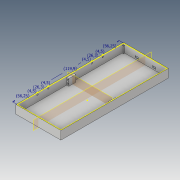
# Autodesk Inventor part: Case Board
Saved by Autodesk Inventor 2019 (Build 230136000, 136)
## iProperties
Created: 2020-09-15
Part Number: Case Board
Material: Generic
Document SubType Name: Modeling
Designer: giacomo
Density: 1 g/cm^3
Appearance: Default
Author: giacomo
Autodesk Inventor part; units mm, degrees
ref_plane "YZ Plane" through (0, 0, 0) normal (1, 0, 0) x (0, 1, 0)
ref_plane "XZ Plane" through (0, 0, 0) normal (0, 1, 0) x (-1, 0, 0)
ref_plane "XY Plane" through (0, 0, 0) normal (0, 0, 1) x (1, 0, 0)
sketch "Sketch1" plane through (0, 0, 0) normal (0, 1, 0) x (-1, 0, 0)
  line L0 (80.1493, 105.9266) -> (-24.8507, 105.9266) construction
  line L1 (-24.8507, 105.9266) -> (-24.8507, -189.0734) construction
  line L2 (-24.8507, -189.0734) -> (80.1493, -189.0734) construction
  line L3 (80.1493, -189.0734) -> (80.1493, 105.9266) construction
  line L4 (80.1493, 91.9266) -> (83.1493, 91.9266) construction
  line L5 (83.1493, 91.9266) -> (83.1493, 84.3266) construction
  line L6 (83.1493, 84.3266) -> (80.1493, 84.3266) construction
  line L7 (80.1493, 84.3266) -> (80.1493, 91.9266) construction
  point P0 (0, 0)
  dimension "d0" = 295
  dimension "d1" = 105
  dimension "d2" = 7.6
  dimension "d3" = 3
  dimension "d4" = 14
  constraints: 16 end point, 4 parallel, 2 horizontal, 2 perpendicular, 1 point on line
  measures "d0" distance of L2.end L0.start
  measures "d1" distance of L1.end L2.end
  measures "d2" distance of L4.end L5.end
  measures "d3" distance of L5.end L6.end
  measures "d4" distance between parallel lines of L0 L4
sketch "Sketch2" plane through (0, 0, 0) normal (0, 1, 0) x (-1, 0, 0)
  line L0 (80.1493, -189.0734) -> (80.1493, 105.9266) construction
  line L1 (-24.8507, -189.0734) -> (80.1493, -189.0734) construction
  line L2 (-24.8507, 105.9266) -> (-24.8507, -189.0734) construction
  line L3 (80.1493, 105.9266) -> (-24.8507, 105.9266) construction
  line L4 (90.1493, 109.9266) -> (90.1493, -193.0734)
  line L5 (-34.8507, -193.0734) -> (-34.8507, 109.9266)
  line L6 (90.1493, 109.9266) -> (-34.8507, 109.9266)
  line L7 (90.1493, -193.0734) -> (-34.8507, -193.0734)
  line L8 (91.6493, -194.5734) -> (91.6493, 111.4266)
  line L9 (91.6493, 111.4266) -> (-36.3507, 111.4266)
  line L10 (-36.3507, 111.4266) -> (-36.3507, -194.5734)
  line L11 (-36.3507, -194.5734) -> (91.6493, -194.5734)
  dimension "d71" = 10
  dimension "d72" = 4
  dimension "d73" = 10
  dimension "d74" = 4
  dimension "d75" = 1.5
  constraints: 16 end point, 2 parallel, 2 perpendicular, 3 other
  measures "d71" distance between parallel lines of L0 L4
  measures "d72" distance between parallel lines of L6 L3
  measures "d73" distance between parallel lines of L2 L5
  measures "d74" distance between parallel lines of L1 L7
  measures "d75" distance between parallel lines of L4 L8
extrude "Extrusion1" add sketch "Sketch2" against normal blind 1 contours L4 L7 L5 L6
extrude "Extrusion2" add sketch "Sketch2" along normal blind 23 and the other way blind 1
sketch "Sketch5" plane through (-91.6493, -1, 111.4266) normal (-1, 0, 0) x (0, 0, 1)
  circle A0 centre (-246, 19) radius 2.25
  circle A1 centre (-90.8, 19) radius 2.25
  circle A2 centre (-215.2, 19) radius 2.25
  circle A3 centre (-60, 19) radius 2.25
  line L0 (0, 0) -> (0, 24) projected
  line L1 (-306, 24) -> (0, 24) projected
  line L2 (-306, 24) -> (-306, 0) projected
  line L3 (0, 0) -> (-306, 0) projected
  point P0 (-111.4266, 1)
  dimension "d35" = 4.5
  dimension "d37" = 4.5
  dimension "d39" = 4.5
  dimension "d40" = 0
  dimension "d41" = 30.8
  dimension "d45" = 4.5
  dimension "d46" = 0
  dimension "d47" = 30.8
  dimension "d76" = 60
  dimension "d77" = 60
  dimension "d144" = 5
  dimension "d145" = 5
  constraints: 4 centre point
  measures "d35" diameter of A0
  measures "d37" diameter of A1
  measures "d39" diameter of A2
  measures "d40" vertical distance of A2.centre A0.centre
  measures "d41" distance of A2.centre A0.centre
  measures "d45" diameter of A3
  measures "d46" vertical distance of A3.centre A1.centre
  measures "d47" distance of A3.centre A1.centre
  measures "d76" distance from line of L2 A0.centre
  measures "d77" distance from line of L0 A3.centre
  measures "d144" distance from line of L1 A2.centre
  measures "d145" distance from line of L1 A1.centre
extrude "Extrusion4" cut sketch "Sketch5" against normal up to surface (1.5 mm away) contours A0 | A1 | A2 | A3
sketch "Sketch7" plane through (-90.1493, 0, -193.0734) normal (1, 0, 0) x (0, 0, -1)
  line L0 (-151.5, 23) -> (-151.5, 0) construction
  line L1 (-141.5, 19) -> (-141.5, 0)
  line L2 (-161.5, 19) -> (-161.5, 0)
  line L3 (-303, 23) -> (0, 23) projected
  line L4 (-303, 0) -> (0, 0) projected
  line L5 (0, 23) -> (0, 0) projected
  line L6 (-161.5, 19) -> (-141.5, 19)
  point P0 (-141.5, 23)
  point P1 (-161.5, 23)
  dimension "d106" = 10
  dimension "d107" = 10
  dimension "d148" = 151.5
  dimension "d149" = 151.5
  dimension "d193" = 19
  constraints: 8 end point, 1 perpendicular
  measures "d106" distance between parallel lines of L1 L0
  measures "d107" distance between parallel lines of L2 L0
  measures "d148" distance from line of L3.start L0
  measures "d149" distance between parallel lines of L5 L0
  measures "d193" distance between parallel lines of L4 L6
extrude "Extrusion6" add sketch "Sketch7" along normal blind 6
ref_plane "Work Plane2" through (-27.6493, 0, 109.9266) normal (1, 0, 0) x (0, 0, -1)
ref_plane "Work Plane4" through (-90.1493, 0, -41.5734) normal (0, 0, 1) x (1, 0, 0)
sketch "Sketch16" plane through (-90.1493, 0, -31.5734) normal (0, 0, 1) x (1, 0, 0)
  line L0 (0, 0) -> (0, 19) projected
  line L1 (0, 19) -> (6, 19) projected
  point P0 (90.1493, 0)
  point P1 (3.5, 14)
  dimension "d108" = 3.5
  dimension "d194" = 5
  measures "d108" distance from line of L0 point (3.5, 14)
  measures "d194" distance from line of L1 point (3.5, 14)
hole "Hole3" at (-86.6493, 14, -31.5734) direction (0, 0, -1) diameter 2.6 depth 5 countersink diameter 5 countersink angle 82
sketch "Sketch17" plane through (-86.6493, 14, -36.5734) normal (0, 0, 1) x (1, 0, 0)
  circle A0 centre (0, 0) radius 1.3 projected
  point P0 (86.6493, -14)
  constraints: 1 coincident
hole "Hole4" at (-86.6493, 14, -36.5734) direction (0, 0, -1) diameter 2.6 depth 15 tip angle 118
sketch "Sketch18" plane through (-90.1493, 0, -31.5734) normal (0, 0, 1) x (1, 0, 0)
  line L0 (0, 0) -> (0, 19) projected
  line L1 (6, 0) -> (0, 0) projected
  point P0 (90.1493, 0)
  point P1 (3.5, 5)
  point P2 (0, 18)
  point P3 (0, 23)
  dimension "d124" = 3.5
  dimension "d125" = 5
  measures "d124" distance from line of L0 point (3.5, 5)
  measures "d125" distance from line of L1 point (3.5, 5)
hole "Hole5" at (-86.6493, 5, -31.5734) direction (0, 0, -1) diameter 2.6 depth 5 countersink diameter 5 countersink angle 82
sketch "Sketch19" plane through (-86.6493, 5, -36.5734) normal (0, 0, 1) x (1, 0, 0)
  circle A0 centre (0, 0) radius 1.3 projected
  point P0 (86.6493, -5)
  constraints: 1 coincident
hole "Hole6" at (-86.6493, 5, -36.5734) direction (0, 0, -1) diameter 2.6 depth 15 tip angle 118
mirror "Mirror6" about plane through (-27.6493, 0, 109.9266) normal (1, 0, 0) of "Extrusion6", "Hole3", "Hole5", "Hole4", "Hole6"
sketch "Sketch23" plane through (0, 0, 0) normal (0, 1, 0) x (1, 0, 0)
  line L0 (-90.1493, 193.0734) -> (34.8507, 193.0734) projected
  line L1 (34.8507, 193.0734) -> (30.8507, 193.0734)
  line L2 (30.8507, 193.0734) -> (30.8507, 189.0734)
  line L3 (30.8507, 189.0734) -> (34.8507, 189.0734)
  line L4 (34.8507, 189.0734) -> (34.8507, 193.0734)
  circle A0 centre (32.8507, 191.0734) radius 1.1
  line L5 (-90.1493, 193.0734) -> (-86.1493, 193.0734)
  line L6 (-86.1493, 193.0734) -> (-86.1493, 189.0734)
  line L7 (-86.1493, 189.0734) -> (-90.1493, 189.0734)
  line L8 (-90.1493, 189.0734) -> (-90.1493, 193.0734)
  circle A1 centre (-88.1493, 191.0734) radius 1.1
  line L9 (34.8507, -109.9687) -> (30.8507, -109.9687)
  line L10 (30.8507, -109.9687) -> (30.8507, -105.9687)
  line L11 (30.8507, -105.9687) -> (34.8507, -105.9687)
  line L12 (34.8507, -105.9687) -> (34.8507, -109.9687)
  circle A2 centre (32.8507, -107.9687) radius 1.1
  line L13 (34.8507, -109.9266) -> (-90.1493, -109.9266) projected
  line L14 (-90.1493, -109.9266) -> (-86.1493, -109.9266)
  line L15 (-86.1493, -109.9266) -> (-86.1493, -105.9266)
  line L16 (-86.1493, -105.9266) -> (-90.1493, -105.9266)
  line L17 (-90.1493, -105.9266) -> (-90.1493, -109.9266)
  circle A3 centre (-88.1493, -107.9266) radius 1.1
  point P0 (0, 0)
  dimension "d159" = 4
  dimension "d160" = 4
  dimension "d161" = 2.2
  dimension "d162" = 2
  dimension "d163" = 2
  dimension "d164" = 4
  dimension "d165" = 4
  dimension "d166" = 2.2
  dimension "d167" = 2
  dimension "d168" = 2
  dimension "d169" = 4
  dimension "d170" = 4
  dimension "d171" = 2.2
  dimension "d172" = 2
  dimension "d173" = 2
  dimension "d174" = 4
  dimension "d175" = 4
  dimension "d176" = 2.2
  dimension "d177" = 2
  dimension "d178" = 2
  constraints: 32 end point, 8 parallel, 4 centre point, 4 horizontal, 4 perpendicular
  measures "d159" distance of L3.end L2.end
  measures "d160" distance of L2.end L1.end
  measures "d161" diameter of A0
  measures "d162" distance from line of L3 A0.centre
  measures "d163" distance from line of L2 A0.centre
  measures "d164" distance of L6.end L7.end
  measures "d165" distance of L5.end L6.end
  measures "d166" diameter of A1
  measures "d167" distance from line of L7 A1.centre
  measures "d168" distance from line of A1.centre L8
  measures "d169" distance of L10.end L11.end
  measures "d170" distance of L9.end L10.end
  measures "d171" diameter of A2
  measures "d172" distance from line of L10 A2.centre
  measures "d173" distance from line of L11 A2.centre
  measures "d174" distance of L16.end L15.end
  measures "d175" distance of L15.end L14.end
  measures "d176" diameter of A3
  measures "d177" distance from line of L17 A3.centre
  measures "d178" distance from line of A3.centre L16
extrude "Extrusion14" add sketch "Sketch23" along normal blind 19
sketch "Sketch24" plane through (-90.1493, 23, -193.0734) normal (0, 0, 1) x (1, 0, 0)
  line L0 (34, -14) -> (43, -14)
  line L1 (43, -14) -> (43, -19)
  line L2 (43, -19) -> (34, -19)
  line L3 (34, -19) -> (34, -14)
  line L4 (4, -23) -> (121, -23) projected
  line L5 (4, -23) -> (4, -4) projected
  line L6 (83, -14) -> (92, -14)
  line L7 (92, -14) -> (92, -19)
  line L8 (92, -19) -> (83, -19)
  line L9 (83, -19) -> (83, -14)
  point P0 (90.1493, -23)
  dimension "d181" = 9
  dimension "d182" = 5
  dimension "d183" = 4
  dimension "d184" = 30
  dimension "d187" = 9
  dimension "d188" = 5
  dimension "d189" = 40
  dimension "d190" = 4
  constraints: 16 end point, 4 parallel, 2 horizontal, 2 perpendicular
  measures "d181" distance of L1.end L2.end
  measures "d182" distance of L0.end L1.end
  measures "d183" distance between parallel lines of L4 L2
  measures "d184" distance between parallel lines of L5 L3
  measures "d187" distance of L7.end L8.end
  measures "d188" distance of L6.end L7.end
  measures "d189" distance between parallel lines of L9 L1
  measures "d190" distance between parallel lines of L4 L8
extrude "Extrusion15" cut sketch "Sketch24" against normal through all
sketch "Sketch25" plane through (-90.1493, 0, -41.5734) normal (0, 0, 1) x (1, 0, 0)
  line L0 (169.9232, 195.9359) -> (-46.5393, 195.9359)
  line L1 (-46.5393, 195.9359) -> (-46.5393, -158.6148)
  line L2 (-46.5393, -158.6148) -> (169.9232, -158.6148)
  line L3 (169.9232, -158.6148) -> (169.9232, 195.9359)
  point P0 (90.1493, 0)
  constraints: 8 end point, 2 parallel, 1 horizontal, 1 perpendicular
extrude "Extrusion16" [suppressed]
sketch "Sketch27" plane through (0, 23, 0) normal (0, 1, 0) x (1, 0, 0)
  line L0 (34.8507, 193.0734) -> (34.8507, -109.9266) projected
  line L1 (-90.1493, 193.0734) -> (34.8507, 193.0734) projected
  line L2 (-90.1493, -109.9266) -> (-90.1493, 193.0734) projected
  line L3 (34.8507, -109.9266) -> (-90.1493, -109.9266) projected
  line L4 (-90.1493, 136.8234) -> (-90.1493, 132.3234) projected
  line L5 (-91.6493, 132.3234) -> (-91.6493, 136.8234) projected
  line L6 (-91.6493, 101.5234) -> (-91.6493, 106.0234) projected
  line L7 (-91.6493, -22.8766) -> (-91.6493, -18.3766) projected
  line L8 (-91.6493, -53.6766) -> (-91.6493, -49.1766) projected
  point P0 (0, 0)
  dimension "d196" = 56.25
  dimension "d197" = 4.5
  dimension "d198" = 26.3
  dimension "d199" = 4.5
  dimension "d200" = 119.9
  dimension "d201" = 4.5
  dimension "d202" = 26.3
  dimension "d203" = 4.5
  dimension "d204" = 56.25
  measures "d196" vertical distance of L5.end L1.start
  measures "d197" distance of L5.start L5.end
  measures "d198" distance of L6.end L5.start
  measures "d199" distance of L6.start L6.end
  measures "d200" distance of L7.end L6.start
  measures "d201" distance of L7.start L7.end
  measures "d202" distance of L8.end L7.start
  measures "d203" distance of L8.start L8.end
  measures "d204" vertical distance of L2.start L8.start
body "Solid1"
